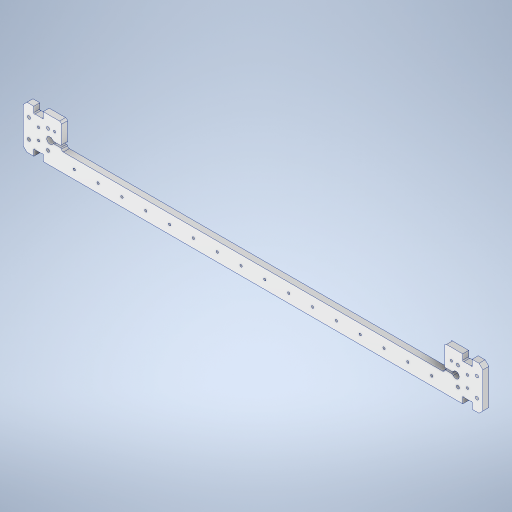
# Autodesk Inventor part: R2 Gantry Bar
Saved by Autodesk Inventor 2024 (Build 280153000, 153)
## iProperties
Created: 2024-08-05
Part Number: R2 Gantry Bar
Material: Aluminum 6061
Document SubType Name: Modeling
Designer: Ishaan
Density: 2.7 g/cm^3
Appearance: Aluminum - Flat
Author: Ishaan
Autodesk Inventor part; units mm, degrees
ref_plane "YZ Plane" through (0, 0, 0) normal (1, 0, 0) x (0, 1, 0)
sketch "Sketch1" plane through (0, 0, 0) normal (0, 0, 1) x (1, 0, 0)
  line L0 (-211.5, -22.7) -> (-238.5, -22.7)
  line L1 (-238.5, -22.7) -> (-238.5, 22.7)
  line L2 (-238.5, 22.7) -> (-211.5, 22.7)
  line L3 (-211.5, 22.7) -> (-211.5, -22.7)
  line L4 (-211.5, -22.7) -> (-238.5, 22.7) construction
  line L5 (-238.5, -22.7) -> (-211.5, 22.7) construction
  line L6 (211.5, -22.7) -> (238.5, -22.7)
  line L7 (238.5, -22.7) -> (238.5, 22.7)
  line L8 (238.5, 22.7) -> (211.5, 22.7)
  line L9 (211.5, 22.7) -> (211.5, -22.7)
  line L10 (211.5, -22.7) -> (238.5, 22.7) construction
  line L11 (238.5, -22.7) -> (211.5, 22.7) construction
  line L12 (-211.5, 2.7) -> (-211.5, 22.7)
  line L13 (211.5, 22.7) -> (211.5, 18.0393)
  line L14 (225, -22.7) -> (-225, -22.7)
  line L15 (-225, -22.7) -> (-225, -3.5)
  line L16 (-225, -3.5) -> (225, -3.5)
  line L17 (225, -3.5) -> (225, -22.7)
  line L18 (225, -22.7) -> (-225, -3.5) construction
  line L19 (-225, -22.7) -> (225, -3.5) construction
  point P0 (0, 0)
  point P1 (0, 0)
  point P2 (-225, 0)
  point P3 (0, -13.1)
  point P4 (-225, 0)
  point P5 (225, 0)
  point P6 (211.5, -3.5)
  point P7 (-211.5, -3.5)
  point P8 (-211.5, -22.7)
  point P9 (211.5, -22.7)
  dimension "d1" = 27
  dimension "d2" = 45.4
  dimension "d97" = 450
  dimension "d98" = 19.2
  constraints: 40 end point, 9 parallel, 5 midpoint, 4 collinear, 3 horizontal, 3 perpendicular, 2 point on line, 1 coincident, 1 horizontal alignment, 1 vertical alignment
  measures "d1" distance of L1.end L2.end
  measures "d2" distance of L0.end L1.end
  measures "d97" distance of L15.end L16.end
  measures "d98" distance between parallel lines of L14 L16
extrude "Extrusion1" add sketch "Sketch1" against normal blind 6.35
sketch "Sketch2" plane through (0, 0, -6.35) normal (0, 0, -1) x (1, 0, 0)
  line L0 (-215, -10) -> (-235, -10) construction
  line L1 (-235, -10) -> (-235, 10) construction
  line L2 (-235, 10) -> (-215, 10) construction
  line L3 (-215, 10) -> (-215, -10) construction
  line L4 (-215, -10) -> (-235, 10) construction
  line L5 (-235, -10) -> (-215, 10) construction
  line L6 (235, -10) -> (215, -10) construction
  line L7 (215, -10) -> (215, 10) construction
  line L8 (215, 10) -> (235, 10) construction
  line L9 (235, 10) -> (235, -10) construction
  line L10 (235, -10) -> (215, 10) construction
  line L11 (215, -10) -> (235, 10) construction
  point P0 (0, 0)
  point P1 (-225, 0)
  point P2 (225, 0)
  point P3 (-225, 0)
  point P4 (225, 0)
  dimension "d8" = 20
  dimension "d9" = 20
  dimension "d10" = 20
  dimension "d11" = 20
  constraints: 24 end point, 10 coincident, 4 midpoint, 4 parallel, 2 horizontal, 2 perpendicular
  measures "d8" distance of L1.end L2.end
  measures "d9" distance of L0.end L1.end
  measures "d10" distance of L7.end L8.end
  measures "d11" distance of L6.end L7.end
hole "Hole1" at (-235, -10, -6.35) at (-215, -10, -6.35) at (-215, 10, -6.35) at (-235, 10, -6.35) at (215, -10, -6.35) at (235, -10, -6.35) at (235, 10, -6.35) at (215, 10, -6.35) direction (0, 0, 1) diameter 3.3 end through all
sketch "Sketch3" plane through (0, 0, -6.35) normal (0, 0, -1) x (1, 0, 0)
  circle A0 centre (215, -10) radius 1.65 projected
  circle A1 centre (235, -10) radius 1.65 projected
  circle A2 centre (235, 10) radius 1.65 projected
  circle A3 centre (215, 10) radius 1.65 projected
  circle A4 centre (-235, -10) radius 1.65 projected
  circle A5 centre (-215, -10) radius 1.65 projected
  circle A6 centre (-215, 10) radius 1.65 projected
  circle A7 centre (-235, 10) radius 1.65 projected
  line L0 (-238.5, 22.7) -> (-238.5, -22.7) projected
  line L1 (-211.5, -22.7) -> (-211.5, 3.5) projected
  line L2 (211.5, 3.5) -> (211.5, -22.7) projected
  line L3 (238.5, -22.7) -> (238.5, 22.7) projected
  line L4 (-238.5, -22.7) -> (-211.5, -22.7) projected
  line L5 (215, 10) -> (235, -10) construction
  line L6 (241.2, 22.7) -> (208.8, 22.7)
  line L7 (208.8, 22.7) -> (208.8, -22.7)
  line L8 (208.8, -22.7) -> (241.2, -22.7)
  line L9 (241.2, -22.7) -> (241.2, 22.7)
  line L10 (241.2, 22.7) -> (208.8, -22.7) construction
  line L11 (208.8, 22.7) -> (241.2, -22.7) construction
  line L12 (238.5, 22.7) -> (-238.5, 22.7) projected
  line L13 (211.5, -22.7) -> (238.5, -22.7) projected
  line L14 (-211.5, 3.5) -> (211.5, 3.5) projected
  line L15 (241.2, -16.2) -> (208.8, -16.2)
  line L16 (208.8, -16.2) -> (208.8, 16.2)
  line L17 (208.8, 16.2) -> (241.2, 16.2)
  line L18 (241.2, 16.2) -> (241.2, -16.2)
  line L19 (241.2, -16.2) -> (208.8, 16.2) construction
  line L20 (208.8, -16.2) -> (241.2, 16.2) construction
  line L21 (-241.2, 22.7) -> (-208.8, 22.7)
  line L22 (-208.8, 22.7) -> (-208.8, -22.7)
  line L23 (-208.8, -22.7) -> (-241.2, -22.7)
  line L24 (-241.2, -22.7) -> (-241.2, 22.7)
  line L25 (-241.2, 22.7) -> (-208.8, -22.7) construction
  line L26 (-208.8, 22.7) -> (-241.2, -22.7) construction
  line L27 (-241.2, 16.2) -> (-208.8, 16.2)
  line L28 (-208.8, 16.2) -> (-208.8, -16.2)
  line L29 (-208.8, -16.2) -> (-241.2, -16.2)
  line L30 (-241.2, -16.2) -> (-241.2, 16.2)
  line L31 (-241.2, 16.2) -> (-208.8, -16.2) construction
  line L32 (-208.8, 16.2) -> (-241.2, -16.2) construction
  point P0 (0, 0)
  point P1 (225, 0)
  point P2 (238.5, 22.7)
  point P3 (211.5, -16.2)
  point P4 (208.8, 3.5)
  point P5 (208.8, 22.7)
  point P6 (-225, 0)
  point P7 (225, -16.2)
  point P8 (-241.2, -16.2)
  point P9 (-238.5, -16.2)
  point P10 (-238.5, 16.2)
  point P11 (-241.2, 16.2)
  point P12 (-211.5, -22.7)
  point P13 (-208.8, 3.5)
  point P14 (238.5, -16.2)
  point P15 (241.2, -16.2)
  point P16 (241.2, 16.2)
  point P17 (238.5, 16.2)
  point P18 (228.8, 22.7)
  point P19 (228.8, -22.7)
  point P20 (221.2, -22.7)
  point P21 (238.5, 22.7)
  point P22 (-208.8, 22.7)
  point P23 (-221.2, -22.7)
  point P24 (-228.8, -22.7)
  point P25 (-228.8, 22.7)
  point P26 (208.8, -16.2)
  point P27 (-238.5, 22.7)
  point P28 (-238.5, -22.7)
  dimension "d100" = 32.4
  dimension "d102" = 6.2
  dimension "d103" = 6.2
  constraints: 50 end point, 10 midpoint, 8 parallel, 4 perpendicular, 3 collinear, 3 horizontal, 3 point on line
  measures "d100" distance between parallel lines of L17 L15
  measures "d102" distance from line of L17 A2.centre
  measures "d103" distance from line of L18 A2.centre
extrude "Extrusion8" add sketch "Sketch3" against normal up to surface (6.35 mm away) contours L0 L27 L24 L21 | L0 L29 L24 L27 | L0 L23 L24 L29 | L29 L22 L23 L1 | L1 L14 L22 L29 | L6 L9 L17 L3 | L14 L2 L15 L7 | L17 L9 L15 L3 | L15 L2 L8 L7 | L15 L9 L8 L3
sketch "Sketch4" plane through (0, 0, -6.35) normal (0, 0, -1) x (1, 0, 0)
  circle A0 centre (215, -10) radius 1.65 construction
  circle A1 centre (235, -10) radius 1.65 construction
  circle A2 centre (235, 10) radius 1.65 construction
  circle A3 centre (215, 10) radius 1.65 construction
  circle A4 centre (-235, -10) radius 1.65 construction
  circle A5 centre (-215, -10) radius 1.65 construction
  circle A6 centre (-215, 10) radius 1.65 construction
  circle A7 centre (-235, 10) radius 1.65 construction
  line L0 (-208.8, -22.7) -> (-208.8, 3.5) construction
  line L1 (-208.8, 3.5) -> (208.8, 3.5) construction
  line L2 (208.8, 3.5) -> (208.8, -22.7) construction
  line L3 (208.8, -22.7) -> (241.2, -22.7) construction
  line L4 (241.2, -22.7) -> (241.2, 22.7) construction
  line L5 (-241.2, 22.7) -> (-241.2, -22.7) construction
  line L6 (208.8, 3.5) -> (-208.8, 3.5) construction
  line L7 (-208.8, 3.5) -> (-208.8, 23.5) construction
  line L8 (-208.8, 23.5) -> (208.8, 23.5) construction
  line L9 (208.8, 23.5) -> (208.8, 3.5) construction
  line L10 (187.5, 13.5) -> (-187.5, 13.5) construction
  line L11 (-241.2, -22.7) -> (-208.8, -22.7) projected
  line L12 (241.2, 22.7) -> (-241.2, 22.7) projected
  point P0 (162.5, 13.5)
  point P1 (137.5, 13.5)
  point P2 (112.5, 13.5)
  point P3 (87.5, 13.5)
  point P4 (62.5, 13.5)
  point P5 (37.5, 13.5)
  point P6 (12.5, 13.5)
  point P7 (-12.5, 13.5)
  point P8 (-37.5, 13.5)
  point P9 (-62.5, 13.5)
  point P10 (-87.5, 13.5)
  point P11 (-112.5, 13.5)
  point P12 (-137.5, 13.5)
  point P13 (-162.5, 13.5)
  point P14 (0, 13.5)
  point P15 (0, 3.5)
  point P16 (-208.8, 13.5)
  dimension "d108" = 25
  constraints: 10 end point, 3 equal length, 3 midpoint, 2 horizontal, 1 horizontal alignment, 1 perpendicular, 1 vertical alignment, 15 other
  measures "d108" distance of L10.start point (162.5, 13.5)
hole "Hole2" at (-187.5, -13.5, -6.35) at (-162.5, -13.5, -6.35) at (-137.5, -13.5, -6.35) at (-112.5, -13.5, -6.35) at (-87.5, -13.5, -6.35) at (-62.5, -13.5, -6.35) at (-37.5, -13.5, -6.35) at (-12.5, -13.5, -6.35) at (12.5, -13.5, -6.35) at (37.5, -13.5, -6.35) at (62.5, -13.5, -6.35) at (87.5, -13.5, -6.35) at (112.5, -13.5, -6.35) at (137.5, -13.5, -6.35) at (162.5, -13.5, -6.35) at (187.5, -13.5, -6.35) direction (0, 0, 1) diameter 2.459 end through all thread size "M3x0.5" class "6H" standard "ANSI Metric M Profile"
sketch "Sketch5" plane through (0, 0, -6.35) normal (0, 0, -1) x (1, 0, 0)
  circle A0 centre (215, -10) radius 1.65 projected
  circle A1 centre (235, -10) radius 1.65 projected
  circle A2 centre (235, 10) radius 1.65 projected
  circle A3 centre (215, 10) radius 1.65 projected
  circle A4 centre (-235, -10) radius 1.65 projected
  circle A5 centre (-215, -10) radius 1.65 projected
  circle A6 centre (-215, 10) radius 1.65 projected
  circle A7 centre (-235, 10) radius 1.65 projected
  line L0 (201, 0) -> (213, 0) construction
  line L1 (201, -1) -> (213, -1)
  line L2 (213, 1) -> (201, 1)
  arc A8 (201, 1) -> (201, -1) centre (201, 0) ccw
  arc A9 (213, -1) -> (213, 1) centre (213, 0) ccw
  circle A10 centre (213, 0) radius 3.5
  circle A11 centre (187.5, 13.5) radius 1.2295 projected
  circle A12 centre (187.5, 13.5) radius 1.2295 projected
  circle A13 centre (162.5, 13.5) radius 1.2295 projected
  circle A14 centre (137.5, 13.5) radius 1.2295 projected
  circle A15 centre (112.5, 13.5) radius 1.2295 projected
  circle A16 centre (87.5, 13.5) radius 1.2295 projected
  circle A17 centre (62.5, 13.5) radius 1.2295 projected
  circle A18 centre (37.5, 13.5) radius 1.2295 projected
  circle A19 centre (12.5, 13.5) radius 1.2295 projected
  circle A20 centre (-12.5, 13.5) radius 1.2295 projected
  circle A21 centre (-37.5, 13.5) radius 1.2295 projected
  circle A22 centre (-62.5, 13.5) radius 1.2295 projected
  circle A23 centre (-87.5, 13.5) radius 1.2295 projected
  circle A24 centre (-112.5, 13.5) radius 1.2295 projected
  circle A25 centre (-137.5, 13.5) radius 1.2295 projected
  circle A26 centre (-162.5, 13.5) radius 1.2295 projected
  circle A27 centre (-187.5, 13.5) radius 1.2295 projected
  circle A28 centre (215, -10) radius 1.65 projected
  circle A29 centre (235, -10) radius 1.65 projected
  circle A30 centre (235, 10) radius 1.65 projected
  circle A31 centre (215, 10) radius 1.65 projected
  circle A32 centre (-235, -10) radius 1.65 projected
  circle A33 centre (-215, -10) radius 1.65 projected
  circle A34 centre (-215, 10) radius 1.65 projected
  circle A35 centre (-235, 10) radius 1.65 projected
  line L3 (-208.8, -22.7) -> (-208.8, 3.5) projected
  line L4 (-208.8, 3.5) -> (208.8, 3.5) projected
  line L5 (208.8, 3.5) -> (208.8, -22.7) projected
  line L6 (208.8, -22.7) -> (241.2, -22.7) projected
  line L7 (241.2, -22.7) -> (241.2, 22.7) projected
  line L8 (-241.2, 22.7) -> (-241.2, -22.7) projected
  line L9 (208.8, -22.7) -> (201, -22.7)
  line L10 (201, -22.7) -> (201, 3.5)
  line L11 (201, 3.5) -> (208.8, 3.5)
  line L12 (208.8, 3.5) -> (208.8, -22.7)
  line L13 (-241.2, -22.7) -> (-208.8, -22.7) projected
  line L14 (241.2, 22.7) -> (-241.2, 22.7) projected
  point P0 (0, 0)
  point P1 (207, 0)
  point P2 (209.6459, 1)
  point P3 (209.6459, -1)
  point P4 (225, 0)
  dimension "d46" = 2
  dimension "d48" = 7
  dimension "d49" = 12
  dimension "d113" = 13.5
  dimension "d114" = 12
  constraints: 16 end point, 4 point on circle, 4 tangent, 3 centre point, 3 parallel, 2 horizontal, 2 point on line, 1 coincident, 1 midpoint, 1 perpendicular
  measures "d46" distance between parallel lines of L1 L2
  measures "d48" diameter of A10
  measures "d49" distance of L0.start L0.end
  measures "d113" distance from line of L0 A11.centre
  measures "d114" distance of L0.end point (225, 0)
extrude "Extrusion9" add sketch "Sketch5" against normal up to surface (6.35 mm away) contours L10 L2 L5 L1 | L1 L5 L9 L10 | L10 L4 L5 L2
extrude "Extrusion4" cut sketch "Sketch5" against normal through all contours L10 L2 L5 L1 | A8 L10 | L5 L2 A10 L1 | A10 L2 A9 L1 | L1 A9 L2 A10
fillet "Fillet1" radius 2 2 edges at (209.6459, -1, -3.175) (209.6459, 1, -3.175)
mirror "Mirror1" about plane through (0, 0, 0) normal (1, 0, 0) of "Extrusion4", "Fillet1", "Extrusion9"
sketch "Sketch7" plane through (0, 0, -6.35) normal (0, 0, -1) x (1, 0, 0)
  arc A0 (-208.3902, -1) -> (-210.0665, -1.9091) centre (-208.3902, -3) ccw projected
  arc A1 (-210.0665, 1.9091) -> (-210.0665, -1.9091) centre (-213, 0) ccw projected
  arc A2 (-210.0665, 1.9091) -> (-208.3902, 1) centre (-208.3902, 3) ccw projected
  line L0 (-208.3902, 1) -> (-201, 1) projected
  line L1 (201, 1) -> (208.3902, 1) projected
  arc A3 (208.3902, 1) -> (210.0665, 1.9091) centre (208.3902, 3) ccw projected
  arc A4 (210.0665, -1.9091) -> (210.0665, 1.9091) centre (213, 0) ccw projected
  arc A5 (210.0665, -1.9091) -> (208.3902, -1) centre (208.3902, -3) ccw projected
  line L2 (208.3902, -1) -> (201, -1) projected
  line L3 (-201, -1) -> (-208.3902, -1) projected
  circle A6 centre (215, -10) radius 1.65 projected
  circle A7 centre (235, -10) radius 1.65 projected
  circle A8 centre (235, 10) radius 1.65 projected
  circle A9 centre (215, 10) radius 1.65 projected
  circle A10 centre (-235, -10) radius 1.65 projected
  circle A11 centre (-215, -10) radius 1.65 projected
  circle A12 centre (-215, 10) radius 1.65 projected
  circle A13 centre (-235, 10) radius 1.65 projected
  line L4 (-201, 3.5) -> (-201, 1) projected
  line L5 (-201, 3.5) -> (201, 3.5) projected
  line L6 (201, 3.5) -> (201, 1) projected
  line L7 (201, -1) -> (201, -22.7) projected
  line L8 (201, -22.7) -> (241.2, -22.7) projected
  line L9 (241.2, -22.7) -> (241.2, 22.7) projected
  line L10 (-241.2, 22.7) -> (-241.2, -22.7) projected
  line L11 (-201, -1) -> (-201, -22.7) projected
  line L12 (220.125, 22.7) -> (229.875, 22.7)
  line L13 (229.875, 22.7) -> (229.875, -22.7)
  line L14 (229.875, -22.7) -> (220.125, -22.7)
  line L15 (220.125, -22.7) -> (220.125, 22.7)
  line L16 (220.125, 22.7) -> (229.875, -22.7) construction
  line L17 (229.875, 22.7) -> (220.125, -22.7) construction
  line L18 (220.125, 16.2) -> (229.875, 16.2)
  line L19 (229.875, 16.2) -> (229.875, -16.2)
  line L20 (229.875, -16.2) -> (220.125, -16.2)
  line L21 (220.125, -16.2) -> (220.125, 16.2)
  line L22 (220.125, 16.2) -> (229.875, -16.2) construction
  line L23 (229.875, 16.2) -> (220.125, -16.2) construction
  line L24 (241.2, 22.7) -> (-241.2, 22.7) projected
  line L25 (-241.2, -22.7) -> (-201, -22.7) projected
  point P0 (0, 0)
  point P1 (225, 0)
  point P2 (225, 16.2)
  point P3 (220.125, -22.7)
  point P4 (220.125, 16.2)
  point P5 (220.125, 1.5762)
  point P6 (220.125, -1.5762)
  point P7 (229.875, 22.7)
  dimension "d117" = 9.75
  dimension "d118" = 32.4
  constraints: 24 end point, 5 midpoint, 4 parallel, 2 horizontal, 2 perpendicular, 1 collinear, 1 point on line
  measures "d117" distance of L13.end L14.end
  measures "d118" distance from line of point (225, 16.2) L20
extrude "Extrusion5" cut sketch "Sketch7" against normal up to surface (6.35 mm away) contours L12 L13 L18 L15 | L20 L13 L8 L15
mirror "Mirror2" about plane through (0, 0, 0) normal (1, 0, 0) of "Extrusion5"
sketch "Sketch8" plane through (0, 0, -6.35) normal (0, 0, -1) x (1, 0, 0)
  line L0 (241.2, -22.7) -> (241.2, 22.7) projected
  line L1 (201, 1) -> (208.3902, 1) projected
  arc A0 (208.3902, 1) -> (210.0665, 1.9091) centre (208.3902, 3) ccw projected
  arc A1 (210.0665, -1.9091) -> (210.0665, 1.9091) centre (213, 0) ccw projected
  arc A2 (210.0665, -1.9091) -> (208.3902, -1) centre (208.3902, -3) ccw projected
  line L2 (208.3902, -1) -> (201, -1) projected
  line L3 (-201, -1) -> (-208.3902, -1) projected
  arc A3 (-208.3902, -1) -> (-210.0665, -1.9091) centre (-208.3902, -3) ccw projected
  arc A4 (-210.0665, 1.9091) -> (-210.0665, -1.9091) centre (-213, 0) ccw projected
  arc A5 (-210.0665, 1.9091) -> (-208.3902, 1) centre (-208.3902, 3) ccw projected
  line L4 (-208.3902, 1) -> (-201, 1) projected
  circle A6 centre (-235, 10) radius 1.65 projected
  circle A7 centre (-215, 10) radius 1.65 projected
  circle A8 centre (-215, -10) radius 1.65 projected
  circle A9 centre (-235, -10) radius 1.65 projected
  circle A10 centre (215, 10) radius 1.65 projected
  circle A11 centre (235, 10) radius 1.65 projected
  circle A12 centre (235, -10) radius 1.65 projected
  circle A13 centre (215, -10) radius 1.65 projected
  circle A14 centre (229.3625, -16.6) radius 0.75
  line L5 (-229.875, 16.2) -> (-229.875, 22.7) projected
  line L6 (-229.875, 22.7) -> (-241.2, 22.7) projected
  line L7 (-241.2, 22.7) -> (-241.2, -22.7) projected
  line L8 (-241.2, -22.7) -> (-229.875, -22.7) projected
  line L9 (-220.125, -16.2) -> (-220.125, -22.7) projected
  line L10 (-220.125, -22.7) -> (-201, -22.7) projected
  line L11 (-201, -1) -> (-201, -22.7) projected
  line L12 (-201, 3.5) -> (-201, 1) projected
  line L13 (-201, 3.5) -> (201, 3.5) projected
  line L14 (201, 3.5) -> (201, 1) projected
  line L15 (201, -1) -> (201, -22.7) projected
  line L16 (201, -22.7) -> (220.125, -22.7) projected
  line L17 (220.125, -22.7) -> (220.125, -16.2) projected
  line L18 (229.875, -16.2) -> (229.875, -22.7) projected
  line L19 (229.875, -22.7) -> (241.2, -22.7) projected
  line L20 (241.2, 22.7) -> (229.875, 22.7) projected
  line L21 (220.125, 22.7) -> (-220.125, 22.7) projected
  line L22 (220.125, -16.2) -> (229.875, -16.2) projected
  line L23 (229.875, 22.7) -> (229.875, 16.2) projected
  line L24 (229.875, 16.2) -> (220.125, 16.2) projected
  line L25 (220.125, 16.2) -> (220.125, 22.7) projected
  line L26 (-220.125, 22.7) -> (-220.125, 16.2) projected
  line L27 (-220.125, 16.2) -> (-229.875, 16.2) projected
  line L28 (-229.875, -22.7) -> (-229.875, -16.2) projected
  line L29 (-229.875, -16.2) -> (-220.125, -16.2) projected
  point P0 (0, 0)
  dimension "d77" = 1.5
  constraints: 1 centre point
  measures "d77" diameter of A14
extrude "Extrusion7" cut sketch "Sketch8" against normal through all contours L18 L22 A14 | A14 L22 L18 | A6 | A7 | A8 | A9 | A10 | A11 | A12 | A13
ref_plane "Work Plane1" through (225, 16.2, -6.35) normal (1, 0, 0) x (0, 0, -1)
mirror "Mirror3" about plane through (225, 16.2, -6.35) normal (1, 0, 0) of "Extrusion7"
ref_plane "Work Plane2" through (220.125, 0, -6.35) normal (0, -1, 0) x (1, 0, 0)
mirror "Mirror4" about plane through (220.125, 0, -6.35) normal (0, -1, 0) of "Extrusion7", "Mirror3"
mirror "Mirror5" about plane through (0, 0, 0) normal (1, 0, 0) of "Extrusion7", "Mirror3", "Mirror4"
sketch "Sketch9" plane through (0, 0, 0) normal (0, 0, 1) x (1, 0, 0)
  circle A0 centre (187.5, -13.5) radius 1.2295 projected
  point P0 (0, 0)
  point P1 (208.2, 10.5)
  dimension "d119" = 24
  dimension "d120" = 20.7
  measures "d119" vertical distance of point (208.2, 10.5) A0.centre
  measures "d120" horizontal distance of point (208.2, 10.5) A0.centre
hole "Hole4" at (208.2, 10.5, 0) direction (0, 0, -1) diameter 2.459 end through all thread size "M3x0.5" class "6H" standard "ANSI Metric M Profile"
mirror "Mirror6" about plane through (0, 0, 0) normal (1, 0, 0) of "Hole4"
chamfer "Chamfer1" distance 4 angle 45 4 edges at (-241.2, -22.7, -3.175) (-241.2, 22.7, -3.175) (241.2, -22.7, -3.175) (241.2, 22.7, -3.175)
fillet "Fillet9" radius 2 4 edges at (201, 22.7, -3.175) (201, -3.5, -3.175) (-201, -3.5, -3.175) (-201, 22.7, -3.175)
fillet "Fillet10" radius 1 4 edges at (-201, -1, -3.175) (-201, 1, -3.175) (201, -1, -3.175) (201, 1, -3.175)
sketch "Sketch10" plane through (0, 0, 0) normal (0, 0, 1) x (1, 0, 0)
  line L0 (-225, 6) -> (-225, -6) construction
  point P0 (0, 0)
  point P1 (-225, 0)
  point P2 (-225, 0)
  dimension "d133" = 12
  constraints: 2 end point, 1 coincident, 1 midpoint, 1 vertical
  measures "d133" distance of L0.start L0.end
hole "Hole5" at (-225, 6, 0) at (-225, -6, 0) direction (0, 0, -1) diameter 2.459 end through all thread size "M3x0.5" class "6H" standard "ANSI Metric M Profile"
mirror "Mirror7" about plane through (0, 0, 0) normal (1, 0, 0) of "Hole5"
equation "\"d103\" = d102"
body "Solid1"
